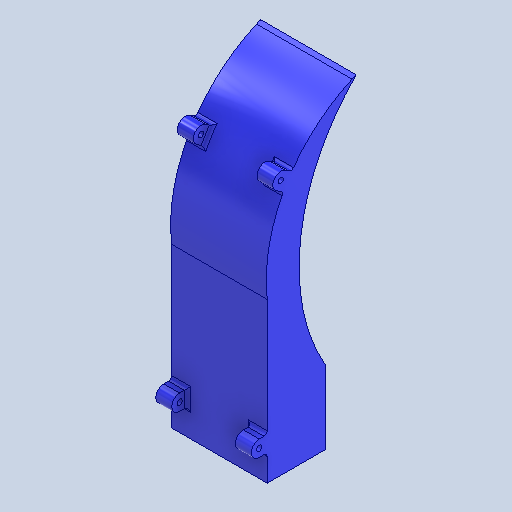
# Autodesk Inventor part: hand-grab-v2-3DP-arm-C
Saved by Autodesk Inventor 2025.1 (Build 291241000, 241)
## iProperties
Created: 2024-10-15
Part Number: hand-grab-v2-3DP-arm-C
Material: ABS プラスチック
Document SubType Name: Modeling
Designer: haruy
Density: 1.06 g/cm^3
Appearance: 青 - 壁塗料 - 光沢
Author: haruy
Autodesk Inventor part; units mm, degrees
ref_plane "YZ Plane" through (0, 0, 0) normal (1, 0, 0) x (0, 1, 0)
ref_plane "XZ Plane" through (0, 0, 0) normal (0, 1, 0) x (-1, 0, 0)
sketch "スケッチ3" plane through (0, 0, 0) normal (1, 0, 0) x (0, 1, 0)
  circle A0 centre (436.4013, 3.8245) radius 122.5
  line L0 (299.9013, 146.3245) -> (303.9013, 146.3245)
  line L1 (303.9013, 146.3245) -> (303.9013, -202.8865)
  line L2 (303.9013, -202.8865) -> (299.9013, -202.8865)
  line L3 (299.9013, -202.8865) -> (299.9013, 146.3245)
  line L4 (436.4013, 3.8245) -> (523.0219, 90.445)
  line L5 (436.4013, 3.8245) -> (436.4013, 126.3245)
  line L6 (436.4013, 3.8245) -> (375.1513, 109.9126)
  line L7 (285.9013, 16.0245) -> (238.1013, 16.0245)
  line L8 (238.1013, 16.0245) -> (238.1013, -8.3755)
  line L9 (238.1013, -8.3755) -> (285.9013, -8.3755)
  line L10 (285.9013, -8.3755) -> (285.9013, 16.0245)
  line L11 (285.9013, 10.3245) -> (288.5013, 10.3245)
  line L12 (288.5013, 10.3245) -> (288.5013, -2.6755)
  line L13 (288.5013, -2.6755) -> (285.9013, -2.6755)
  line L14 (285.9013, -2.6755) -> (285.9013, 10.3245)
  line L15 (288.5013, 6.8245) -> (302.9013, 6.8245)
  line L16 (302.9013, 6.8245) -> (302.9013, 0.8245)
  line L17 (302.9013, 0.8245) -> (288.5013, 0.8245)
  line L18 (288.5013, 0.8245) -> (288.5013, 6.8245)
  line L19 (289.9013, 74.154) -> (285.9013, 74.154)
  line L20 (285.9013, 74.154) -> (285.9013, -68.3086)
  line L21 (285.9013, -68.3086) -> (289.9013, -68.3086)
  line L22 (289.9013, -68.3086) -> (289.9013, 74.154)
  line L23 (299.9013, 12.8245) -> (293.9013, 12.8245)
  line L24 (293.9013, 12.8245) -> (293.9013, -5.1755)
  line L25 (293.9013, -5.1755) -> (299.9013, -5.1755)
  line L26 (299.9013, -5.1755) -> (299.9013, 12.8245)
  line L27 (375.1513, 109.9126) -> (303.9013, 109.9126)
  circle A1 centre (-96.0987, 3.8245) radius 600
  line L28 (303.9013, 146.3245) -> (428.795, 146.3245)
  arc A2 (523.0219, 90.445) -> (428.795, 146.3245) centre (439.4013, 56.8245) ccw
  circle A3 centre (-96.0987, 3.8245) radius 400
  circle A4 centre (302.4013, 137.3245) radius 1.5
  circle A5 centre (302.4013, 119.3245) radius 1.5
  line L29 (303.9013, 109.9126) -> (299.9013, 109.9126)
  line L30 (303.9013, 146.3245) -> (318.9013, 146.3245)
  line L31 (318.9013, 146.3245) -> (318.9013, 109.9126)
  line L32 (318.9013, 109.9126) -> (303.9013, 109.9126)
  line L33 (303.9013, 109.9126) -> (303.9013, 146.3245)
  circle A6 centre (311.4013, 131.3245) radius 1.5
  circle A7 centre (311.4013, 116.3245) radius 1.5
  line L34 (328.9013, 146.3245) -> (328.9013, 109.9126)
  circle A8 centre (501.4013, 128.9702) radius 1.7
  circle A9 centre (350.4013, 151.3245) radius 1.7
  circle A10 centre (501.4013, 128.9702) radius 5
  circle A11 centre (350.4013, 151.3245) radius 5
  line L35 (345.4013, 151.3245) -> (345.4013, 146.3245)
  line L36 (355.4013, 151.3245) -> (355.4013, 146.3245)
  circle A12 centre (335.4013, 151.3245) radius 5
  circle A13 centre (335.4013, 151.3245) radius 1.7
  line L37 (328.9013, 146.3245) -> (328.9013, 156.3245)
  line L38 (328.9013, 156.3245) -> (436.4013, 156.3245)
  circle A14 centre (489.2896, 137.8193) radius 5
  circle A15 centre (489.2896, 137.8193) radius 1.7
  circle A16 centre (103.9013, 3.8245) radius 600
  line L39 (523.0219, 90.445) -> (506.0106, 130.908)
  line L40 (436.4013, 156.3245) -> (490.5132, 142.6673)
  line L41 (492.2393, 141.8565) -> (504.351, 133.0074)
  line L42 (485.1551, 140.631) -> (482.1278, 136.1793)
  line L43 (493.4242, 135.0077) -> (490.6655, 130.9509)
  point P0 (0, 0)
  point P1 (303.9013, 128.1185)
  point P2 (497.234, 131.733)
  point P3 (453.1551, 145.8951)
  point P4 (497.1922, 131.669)
  point P5 (463.1906, 143.7544)
  point P6 (497.2988, 131.8284)
  point P7 (497.321, 131.86)
  point P8 (350.4013, 156.3245)
  point P9 (350.4013, 146.3245)
  point P10 (498.1425, 125.1781)
  point P11 (521.9251, 93.054)
  dimension "d65" = 3
  dimension "d66" = 3
  dimension "d67" = 9
  dimension "d68" = 18
  dimension "d69" = 2.5
  dimension "d70" = 2.5
  dimension "d71" = 15
  dimension "d72" = 0
  dimension "d73" = 3
  dimension "d74" = 3
  dimension "d75" = 15
  dimension "d76" = 15
  dimension "d77" = 7.5
  dimension "d78" = 7.5
  dimension "d79" = 10
  dimension "d80" = 3.4
  dimension "d81" = 3.4
  dimension "d82" = 10
  dimension "d83" = 10
  dimension "d84" = 86
  dimension "d85" = 10
  dimension "d86" = 3.4
  dimension "d87" = 15
  dimension "d88" = 10
  dimension "d89" = 3.4
  dimension "d90" = 15
  dimension "d91" = 65
  constraints: 88 end point, 18 point on circle, 17 centre point, 13 tangent, 5 perpendicular, 5 point on line, 4 coincident, 3 parallel, 2 vertical, 1 horizontal, 1 midpoint
  measures "d65" diameter of A4
  measures "d66" diameter of A5
  measures "d67" distance from line of A4.centre L0
  measures "d68" distance of A5.centre A4.centre
  measures "d69" distance from line of A4.centre L3
  measures "d70" distance from line of A5.centre L3
  measures "d71" distance of L31.end L32.end
  measures "d72" distance between parallel lines of L27 L32
  measures "d73" diameter of A6
  measures "d74" diameter of A7
  measures "d75" distance from line of L30 A6.centre
  measures "d76" distance of A7.centre A6.centre
  measures "d77" distance from line of A7.centre L1
  measures "d78" horizontal distance of A6.centre point (303.901, 128.119)
  measures "d79" distance between parallel lines of L31 L34
  measures "d80" diameter of A8
  measures "d81" diameter of A9
  measures "d82" diameter of A10
  measures "d83" diameter of A11
  measures "d84" horizontal distance of point (436.401, 3.824) A11.centre
  measures "d85" diameter of A12
  measures "d86" diameter of A13
  measures "d87" distance of A12.centre A9.centre
  measures "d88" diameter of A14
  measures "d89" diameter of A15
  measures "d90" distance of A14.centre A8.centre
  measures "d91" horizontal distance of point (436.401, 3.824) A8.centre
extrude "押し出し4" add sketch "スケッチ3" along normal blind 60 contours A0 A1 A2 L39 | A0 L27 L34 L28 A2 A1
extrude "押し出し5" add sketch "スケッチ3" along normal blind 10 contours A2 A14 A1 | A1 A14 L43 A2 | A14 A1 A15 | A1 A15 A14 | A2 L42 A14 | L35 A11 L28 | A11 | L28 A11 L36
fillet "フィレット2" radius 2 6 edges at (10, 350.4013, 146.3245) (5, 345.4013, 146.3245) (5, 355.4013, 146.3245) (5, 482.1278, 136.1793) (5, 490.6655, 130.9509) (10, 486.4693, 133.6838)
ref_plane "作業平面2" through (30, 0, 0) normal (1, 0, 0) x (0, 0, -1)
mirror "ミラー2" about plane through (30, 0, 0) normal (1, 0, 0) of "押し出し5", "フィレット2"
equation "\"d70\" = d69"
equation "\"d78\" = d77"
